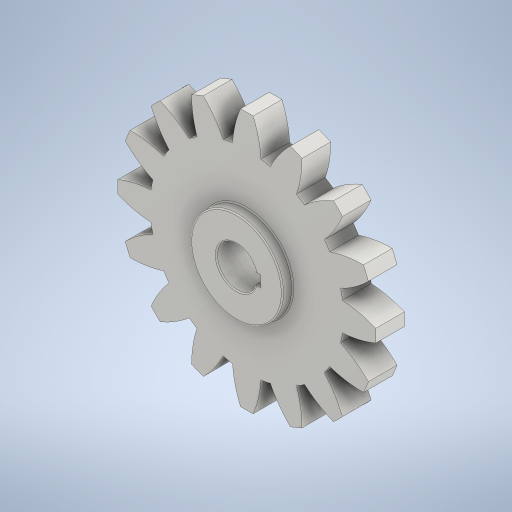
# Autodesk Inventor part: Spur Gear1
Saved by Autodesk Inventor 2024.2 (Build 282272000, 272)
## iProperties
CustomPartVersion: 1
Created: 2024-04-25
Part Number: Spur Gear1
Material: Steel
Document SubType Name: Modeling
Designer: pokla
Categories: <?xml version="1.0" encoding="UTF-16"?> <MemberInstance><Categories><FamilyTemplate><FamilyTemplateParameter ValueType="xs:double" Id="1" ObjectReferenceKey="da_z" ObjectType="kUserParameterObject"/><FamilyTemplateParameter ValueType="xs:double" Id="2" ObjectReferenceKey="da_b" ObjectType="kUserParameterObject"/><FamilyTemplateParameter ValueType="xs:double" Id="3" ObjectReferenceKey="da_beta" ObjectType="kUserParameterObject"/><FamilyTemplateParameter ValueType="xs:double" Id="4" ObjectReferenceKey="da_da" ObjectType="kUserParameterObject"/><FamilyTemplateParameter ValueType="xs:double" Id="5" ObjectReferenceKey="da_aw" ObjectType="kUserParameterObject"/><FamilyTemplateParameter ValueType="xs:string" Id="6" ObjectReferenceKey="EAIAABAAAACIAQAAAAAAAIAAAAAAAAAA" ObjectType="83910656" SubObjectId="SurfaceGeometry"/></FamilyTemplate><ParamToTemplateMap><ParamToTemplate CategoryParameter="//CategoryParameter[@InternalName='046C89C9-8512-4d59-83FE-43B91F4F132A']" TemplateParameter="1"/><ParamToTemplate CategoryParameter="//CategoryParameter[@InternalName='2552DF32-E462-4b46-AEBF-C6C7768E72AC']" TemplateParameter="2"/><ParamToTemplate CategoryParameter="//CategoryParameter[@InternalName='C9EE641D-15FC-4fae-A226-E94C4372FDD7']" TemplateParameter="3"/><ParamToTemplate><ParamToTemplate CategoryParameter="//CategoryParameter[@InternalName='00B6519A-459B-49c7-AD84-2E56D39A5744']" ConstantValue="0.000000"/></ParamToTemplate><ParamToTemplate><ParamToTemplate CategoryParameter="//CategoryParameter[@InternalName='04B31F0E-C7A6-4894-AA32-9629BEFACF47']" ConstantValue="1.000000"/></ParamToTemplate><ParamToTemplate><ParamToTemplate CategoryParameter="//CategoryParameter[@InternalName='43CBEC2E-7847-49e7-A936-2F7889FCB2D9']" ConstantValue="0.250000"/></ParamToTemplate><ParamToTemplate><ParamToTemplate CategoryParameter="//CategoryParameter[@InternalName='B1EFC894-105D-4ebd-86BF-FA20ED196853']" ConstantValue="0.333500"/></ParamToTemplate><ParamToTemplate><ParamToTemplate CategoryParameter="//CategoryParameter[@InternalName='51175063-3D10-4879-93E8-6246FE8B403D']" ConstantValue="2060000000.000000"/></ParamToTemplate><ParamToTemplate><ParamToTemplate CategoryParameter="//CategoryParameter[@InternalName='A3A52E27-4454-46a9-B0BD-C932399B70AF']" ConstantValue="0.300000"/></ParamToTemplate><ParamToTemplate><ParamToTemplate CategoryParameter="//CategoryParameter[@InternalName='91B76062-C214-41d9-B1B9-14D2AB99603D']" ConstantValue="1.250632"/></ParamToTemplate><ParamToTemplate><ParamToTemplate CategoryParameter="//CategoryParameter[@InternalName='374E806E-8B8A-4dda-A9AA-1039D6500AD2']" ConstantValue="0.799596"/></ParamToTemplate><ParamToTemplate><ParamToTemplate CategoryParameter="//CategoryParameter[@InternalName='2D373A89-B862-43d6-8D0B-0CBF12AB9F6C']" ConstantValue="0.253073"/></ParamToTemplate><ParamToTemplate CategoryParameter="//CategoryParameter[@InternalName='37777632-D6A2-4fac-9D53-DB8ACD95C989']" TemplateParameter="4"/><ParamToTemplate CategoryParameter="//CategoryParameter[@InternalName='FD1017F1-B727-4f7e-9707-0F86F1FF9423']" TemplateParameter="5"/><ParamToTemplate><ParamToTemplate CategoryParameter="//CategoryParameter[@InternalName='9E1B4470-B2D3-4ff1-B813-535BB4CDF51A']" ConstantValue="3520000.000000"/></ParamToTemplate><ParamToTemplate><ParamToTemplate CategoryParameter="//CategoryParameter[@InternalName='F8452263-BFF6-458c-9FB1-07C4B99E95CD']" ConstantValue="11400000.000000"/></ParamToTemplate><ParamToTemplate><ParamToTemplate CategoryParameter="//CategoryParameter[@InternalName='3E3BB259-FD49-497f-8171-6EBC954A3479']" ConstantValue="2.000000"/></ParamToTemplate><ParamToTemplate CategoryParameter="//CategoryParameter[@InternalName='27C3BAF2-7550-4e4b-AE2C-0DB134B7D9B7']" TemplateParameter="6"/></ParamToTemplateMap><Category DisplayName="Gear" InternalName="DC85795E-93AB-48d5-8EEE-5A27447B64BD" Mnemonic="Gear"><CategoryParameter DisplayName="z" InternalName="046C89C9-8512-4d59-83FE-43B91F4F132A" Mnemonic="z"/><CategoryParameter DisplayName="b" InternalName="2552DF32-E462-4b46-AEBF-C6C7768E72AC" Mnemonic="b"/><CategoryParameter DisplayName="||b|" InternalName="C9EE641D-15FC-4fae-A226-E94C4372FDD7" Mnemonic="beta"/><CategoryParameter DisplayName="x" InternalName="00B6519A-459B-49c7-AD84-2E56D39A5744" Mnemonic="x"/><CategoryParameter DisplayName="a*" InternalName="04B31F0E-C7A6-4894-AA32-9629BEFACF47" Mnemonic="a"/><CategoryParameter DisplayName="c*" InternalName="43CBEC2E-7847-49e7-A936-2F7889FCB2D9" Mnemonic="c"/><CategoryParameter DisplayName="r|.f|*" InternalName="B1EFC894-105D-4ebd-86BF-FA20ED196853" Mnemonic="rf"/><CategoryParameter DisplayName="E" InternalName="51175063-3D10-4879-93E8-6246FE8B403D" Mnemonic="E"/><CategoryParameter DisplayName="||m|" InternalName="A3A52E27-4454-46a9-B0BD-C932399B70AF" Mnemonic="mi"/><Category DisplayName="SpurGear" InternalName="26C5A22E-A91E-4dfd-A3B3-23CCAFAE1764" Mnemonic="SpurGear"><CategoryParameter DisplayName="m" InternalName="91B76062-C214-41d9-B1B9-14D2AB99603D" Mnemonic="m"/><CategoryParameter DisplayName="P" InternalName="374E806E-8B8A-4dda-A9AA-1039D6500AD2" Mnemonic="PP"/><CategoryParameter DisplayName="||a|" InternalName="2D373A89-B862-43d6-8D0B-0CBF12AB9F6C" Mnemonic="alpha"/><CategoryParameter DisplayName="d|.a|" InternalName="37777632-D6A2-4fac-9D53-DB8ACD95C989" Mnemonic="da"/><CategoryParameter DisplayName="a|.w|" InternalName="FD1017F1-B727-4f7e-9707-0F86F1FF9423" Mnemonic="aw"/><CategoryParameter DisplayName="||s||.Flim|" InternalName="9E1B4470-B2D3-4ff1-B813-535BB4CDF51A" Mnemonic="sFlim"/><CategoryParameter DisplayName="||s||.Hlim|" InternalName="F8452263-BFF6-458c-9FB1-07C4B99E95CD" Mnemonic="sHlim"/><CategoryParameter DisplayName="type" InternalName="3E3BB259-FD49-497f-8171-6EBC954A3479" Mnemonic="type"/><CategoryParameter DisplayName="PitchDiameter" InternalName="27C3BAF2-7550-4e4b-AE2C-0DB134B7D9B7" Mnemonic="IDS_PITCHDIAM"/></Category></Category></Categories></MemberInstance>
Density: 1 g/cm^3
Appearance: Steel
Author: pokla
Autodesk Inventor part; units mm, degrees
sketch "Sketch1" plane through (0, 0, 0) normal (0, 0, 1) x (1, 0, 0)
  circle A0 centre (0, 0) radius 112.5569
  dimension "d0" = 225.1138
  constraints: 1 centre point
  measures "d0" diameter of A0
extrude "Extrusion1" add sketch "Sketch1" along normal blind 25
ref_plane "Work Plane2" through (0, 0, 12.5) normal (0, 0, 1) x (1, 0, 0)
sketch "Sketch2" plane through (0, 0, 0) normal (0, 0, -1) x (-1, 0, 0)
  circle A0 centre (0, 0) radius 112.5569 projected
  circle A1 centre (0, 0) radius 100.0506
  dimension "d3" = 200.1011
  constraints: 1 centre point, 1 coincident
  measures "d3" diameter of A1
surface extrude "Pitch Diameter" sketch "Sketch2" against normal through all shown no curves A1
ref_plane "Work Plane8" through (0, 0, 0) normal (0.9807853, 0.1950903, 0) x (0, 0, 1)
ref_plane "Work Plane9" through (0, 0, 0) normal (1, 0, 0) x (0, 1, 0)
spur gear teeth "Spur Gear" teeth 16 pitch diameter 200.1011 tip diameter 225.1138 root diameter 168.8353 face width 25 start plane through (0, 0, 0) normal (0, 0, -1) x (-1, 0, 0)
sketch "Sketch3" plane through (0, 0, 25) normal (0, 0, 1) x (1, 0, 0)
  arc A0 (-37.9193, 105.9773) -> (-48.1243, 101.7502) centre (0, 0) ccw projected
  arc A1 (-48.1243, 101.7502) -> (-43.3994, 72.4074) centre (43.7364, 101.4903) ccw projected
  arc A2 (-43.3994, 72.4074) -> (-50.2875, 67.8049) centre (0, 0) ccw projected
  arc A3 (-50.2875, 67.8049) -> (-75.5886, 83.3991) centre (-110.502, -1.5685) ccw projected
  arc A4 (-75.5886, 83.3991) -> (-83.3991, 75.5886) centre (0, 0) ccw projected
  arc A5 (-83.3991, 75.5886) -> (-67.8049, 50.2875) centre (1.5685, 110.502) ccw projected
  arc A6 (-67.8049, 50.2875) -> (-72.4074, 43.3994) centre (0, 0) ccw projected
  arc A7 (-72.4074, 43.3994) -> (-101.7502, 48.1243) centre (-101.4903, -43.7364) ccw projected
  arc A8 (-101.7502, 48.1243) -> (-105.9773, 37.9193) centre (0, 0) ccw projected
  arc A9 (-105.9773, 37.9193) -> (-81.8878, 20.5118) centre (-40.8382, 102.6908) ccw projected
  arc A10 (-81.8878, 20.5118) -> (-83.504, 12.3866) centre (0, 0) ccw projected
  arc A11 (-83.504, 12.3866) -> (-112.4213, 5.5229) centre (-77.0276, -79.2458) ccw projected
  arc A12 (-112.4213, 5.5229) -> (-112.4213, -5.5229) centre (0, 0) ccw projected
  arc A13 (-112.4213, -5.5229) -> (-83.504, -12.3866) centre (-77.0276, 79.2458) ccw projected
  arc A14 (-83.504, -12.3866) -> (-81.8878, -20.5118) centre (0, 0) ccw projected
  arc A15 (-81.8878, -20.5118) -> (-105.9773, -37.9193) centre (-40.8382, -102.6908) ccw projected
  arc A16 (-105.9773, -37.9193) -> (-101.7502, -48.1243) centre (0, 0) ccw projected
  arc A17 (-101.7502, -48.1243) -> (-72.4074, -43.3994) centre (-101.4903, 43.7364) ccw projected
  arc A18 (-72.4074, -43.3994) -> (-67.8049, -50.2875) centre (0, 0) ccw projected
  arc A19 (-67.8049, -50.2875) -> (-83.3991, -75.5886) centre (1.5685, -110.502) ccw projected
  arc A20 (-83.3991, -75.5886) -> (-75.5886, -83.3991) centre (0, 0) ccw projected
  arc A21 (-75.5886, -83.3991) -> (-50.2875, -67.8049) centre (-110.502, 1.5685) ccw projected
  arc A22 (-50.2875, -67.8049) -> (-43.3994, -72.4074) centre (0, 0) ccw projected
  arc A23 (-43.3994, -72.4074) -> (-48.1243, -101.7502) centre (43.7364, -101.4903) ccw projected
  arc A24 (-48.1243, -101.7502) -> (-37.9193, -105.9773) centre (0, 0) ccw projected
  arc A25 (-37.9193, -105.9773) -> (-20.5118, -81.8878) centre (-102.6908, -40.8382) ccw projected
  arc A26 (-20.5118, -81.8878) -> (-12.3866, -83.504) centre (0, 0) ccw projected
  arc A27 (-12.3866, -83.504) -> (-5.5229, -112.4213) centre (79.2458, -77.0276) ccw projected
  arc A28 (-5.5229, -112.4213) -> (5.5229, -112.4213) centre (0, 0) ccw projected
  arc A29 (5.5229, -112.4213) -> (12.3866, -83.504) centre (-79.2458, -77.0276) ccw projected
  arc A30 (12.3866, -83.504) -> (20.5118, -81.8878) centre (0, 0) ccw projected
  arc A31 (20.5118, -81.8878) -> (37.9193, -105.9773) centre (102.6908, -40.8382) ccw projected
  arc A32 (37.9193, -105.9773) -> (48.1243, -101.7502) centre (0, 0) ccw projected
  arc A33 (48.1243, -101.7502) -> (43.3994, -72.4074) centre (-43.7364, -101.4903) ccw projected
  arc A34 (43.3994, -72.4074) -> (50.2875, -67.8049) centre (0, 0) ccw projected
  arc A35 (50.2875, -67.8049) -> (75.5886, -83.3991) centre (110.502, 1.5685) ccw projected
  arc A36 (75.5886, -83.3991) -> (83.3991, -75.5886) centre (0, 0) ccw projected
  arc A37 (83.3991, -75.5886) -> (67.8049, -50.2875) centre (-1.5685, -110.502) ccw projected
  arc A38 (67.8049, -50.2875) -> (72.4074, -43.3994) centre (0, 0) ccw projected
  arc A39 (72.4074, -43.3994) -> (101.7502, -48.1243) centre (101.4903, 43.7364) ccw projected
  arc A40 (101.7502, -48.1243) -> (105.9773, -37.9193) centre (0, 0) ccw projected
  arc A41 (105.9773, -37.9193) -> (81.8878, -20.5118) centre (40.8382, -102.6908) ccw projected
  arc A42 (81.8878, -20.5118) -> (83.504, -12.3866) centre (0, 0) ccw projected
  arc A43 (83.504, -12.3866) -> (112.4213, -5.5229) centre (77.0276, 79.2458) ccw projected
  arc A44 (112.4213, -5.5229) -> (112.4213, 5.5229) centre (0, 0) ccw projected
  arc A45 (112.4213, 5.5229) -> (83.504, 12.3866) centre (77.0276, -79.2458) ccw projected
  arc A46 (83.504, 12.3866) -> (81.8878, 20.5118) centre (0, 0) ccw projected
  arc A47 (81.8878, 20.5118) -> (105.9773, 37.9193) centre (40.8382, 102.6908) ccw projected
  arc A48 (105.9773, 37.9193) -> (101.7502, 48.1243) centre (0, 0) ccw projected
  arc A49 (101.7502, 48.1243) -> (72.4074, 43.3994) centre (101.4903, -43.7364) ccw projected
  arc A50 (72.4074, 43.3994) -> (67.8049, 50.2875) centre (0, 0) ccw projected
  arc A51 (67.8049, 50.2875) -> (83.3991, 75.5886) centre (-1.5685, 110.502) ccw projected
  arc A52 (83.3991, 75.5886) -> (75.5886, 83.3991) centre (0, 0) ccw projected
  arc A53 (75.5886, 83.3991) -> (50.2875, 67.8049) centre (110.502, -1.5685) ccw projected
  arc A54 (50.2875, 67.8049) -> (43.3994, 72.4074) centre (0, 0) ccw projected
  arc A55 (43.3994, 72.4074) -> (48.1243, 101.7502) centre (-43.7364, 101.4903) ccw projected
  arc A56 (48.1243, 101.7502) -> (37.9193, 105.9773) centre (0, 0) ccw projected
  arc A57 (37.9193, 105.9773) -> (20.5118, 81.8878) centre (102.6908, 40.8382) ccw projected
  arc A58 (20.5118, 81.8878) -> (12.3866, 83.504) centre (0, 0) ccw projected
  arc A59 (12.3866, 83.504) -> (5.5229, 112.4213) centre (-79.2458, 77.0276) ccw projected
  arc A60 (5.5229, 112.4213) -> (-5.5229, 112.4213) centre (0, 0) ccw projected
  arc A61 (-5.5229, 112.4213) -> (-12.3866, 83.504) centre (79.2458, 77.0276) ccw projected
  arc A62 (-12.3866, 83.504) -> (-20.5118, 81.8878) centre (0, 0) ccw projected
  arc A63 (-20.5118, 81.8878) -> (-37.9193, 105.9773) centre (-102.6908, 40.8382) ccw projected
  circle A64 centre (0, 0) radius 17.5
  dimension "d51" = 35
  constraints: 1 centre point
  measures "d51" diameter of A64
extrude "Extrusion2" cut sketch "Sketch3" against normal through all contours A64
sketch "Sketch5" plane through (0, 0, 25) normal (0, 0, 1) x (1, 0, 0)
  circle A0 centre (0, 0) radius 40
  circle A1 centre (0, 0) radius 17.5
  dimension "d55" = 80
  dimension "d56" = 35
  constraints: 2 centre point, 2 coincident
  measures "d55" diameter of A0
  measures "d56" diameter of A1
extrude "Extrusion3" add sketch "Sketch5" along normal blind 9
sketch "Sketch6" plane through (0, 0, 25) normal (0, 0, 1) x (1, 0, 0)
  line L0 (0, 5) -> (21, 5)
  line L1 (21, 5) -> (21, -5)
  line L2 (21, -5) -> (0, -5)
  line L3 (0, -5) -> (0, 5)
  point P0 (0, 0)
  point P1 (0, 0)
  dimension "d59" = 21
  dimension "d60" = 10
  constraints: 8 end point, 2 parallel, 1 coincident, 1 horizontal, 1 midpoint, 1 perpendicular
  measures "d59" distance of L1.end L2.end
  measures "d60" distance of L0.end L1.end
extrude "Extrusion4" cut sketch "Sketch6" along normal through all both and the other way through all
fillet "Fillet1" radius 1 4 edges at (-17.5, 0, 34) (-40, 0, 34) (-40, 0, 25) (-17.5, 0, 0)
equation "\"d0\" = da_da"
equation "\"d1\" = da_b"
equation "\"d3\" = da_d"
equation "\"d16\" = da_aw"
equation "\"d43\" = da_aw"
equation "\"d46\" = da_aw"
equation "\"da_da\" = 225.11376"
equation "\"da_b\" = 25"
equation "\"da_d\" = 200.10112"
equation "\"da_aw\" = 494"
body "Solid1"
body "Srf1"
